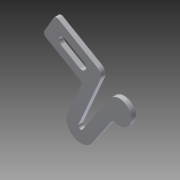
# Autodesk Inventor part: plastic-spring
Saved by Autodesk Inventor 2015 (Build 190159000, 159)
## iProperties
Created: 2014-10-04
Part Number: plastic-spring
Material: ABS Plastic
Document SubType Name: Modeling
Designer: Adam
Density: 1.06 g/cm^3
Appearance: Smooth - White
Author: Adam
Autodesk Inventor part; units mm, degrees
ref_plane "YZ Plane" through (0, 0, 0) normal (1, 0, 0) x (0, 1, 0)
ref_plane "XZ Plane" through (0, 0, 0) normal (0, 1, 0) x (-1, 0, 0)
ref_plane "Work Plane1" through (0, 0, 0.5) normal (0, 0, 1) x (1, 0, 0)
sketch "Sketch1" plane through (0, 0, 0.5) normal (0, 0, 1) x (1, 0, 0)
  line L0 (-82.7297, 47.8765) -> (82.7746, -47.6774) construction
  arc A0 (-7.7942, 4.6125) -> (-6.6121, 9.7651) centre (-15.5885, 9.1125) ccw construction
  arc A1 (-11.6654, 1.0125) -> (-7.7942, 4.6125) centre (-15.5885, 9.1125) ccw construction
  line L1 (-11.2583, 6.6125) -> (-15.5885, 9.1125) construction
  line L2 (-12.6807, 17.8261) -> (-21.6807, 2.2376) construction
  line L3 (-21.3116, 18.0806) -> (-26.3941, 9.2775) construction
  line L4 (-23.2429, 13.5318) -> (-25.2874, 14.7122) construction
  line L5 (-28.644, 9.9991) -> (-48.2897, 21.3415) construction
  line L6 (-42.5297, 31.3181) -> (-22.884, 19.9757) construction
  arc A2 (-28.7943, 15.1203) -> (-27.3943, 17.5452) centre (-28.0943, 16.3328) ccw construction
  line L7 (-27.3943, 17.5452) -> (-32.5904, 20.5452) construction
  arc A3 (-32.5904, 20.5452) -> (-33.9904, 18.1203) centre (-33.2904, 19.3328) ccw construction
  line L8 (-33.9904, 18.1203) -> (-28.7943, 15.1203) construction
  arc A4 (-13.829, 2.4121) -> (-16.4545, 9.6125) centre (-12.1244, 7.1125) ccw
  line L9 (-16.3046, 9.8558) -> (-30.232, -11.3665)
  line L10 (-20.1032, 14.7286) -> (-31.9722, -10.3906)
  arc A5 (-31.9722, -10.3906) -> (-30.232, -11.3665) centre (-31.068, -10.8179) ccw
  arc A6 (-20.1032, 14.7286) -> (-21.3157, 18.6083) centre (-22.8157, 16.0103) ccw
  arc A7 (-28.2563, 9.1773) -> (-28.6605, 10.4705) centre (-29.1605, 9.6045) ccw
  line L11 (-28.2563, 9.1773) -> (-36.4929, -8.2546)
  line L12 (-15.5944, 1.8249) -> (-26.0517, -14.1098)
  line L13 (-29.644, 8.267) -> (-28.644, 9.9991) construction
  line L14 (-15.2247, 16.6235) -> (-28.1306, -5.7301) construction
  arc A8 (-13.829, 2.4121) -> (-15.5944, 1.8249) centre (-14.3403, 1.0019) ccw
  arc A9 (-28.9943, 14.7739) -> (-27.1943, 17.8916) centre (-28.0943, 16.3328) ccw
  line L15 (-28.9943, 14.7739) -> (-36.7885, 19.2739)
  line L16 (-34.9885, 22.3916) -> (-27.1943, 17.8916)
  line L17 (-28.6605, 10.4705) -> (-43.3316, 18.9409)
  line L18 (-43.8807, 20.9899) -> (-40.0207, 27.6756)
  line L19 (-37.9717, 28.2247) -> (-21.3157, 18.6083)
  line L20 (-12.1244, 7.1125) -> (-15.5944, 1.8249) construction
  arc A10 (-36.4929, -8.2546) -> (-26.0517, -14.1098) centre (-31.068, -10.8179) ccw
  arc A11 (-34.9885, 22.3916) -> (-36.7885, 19.2739) centre (-35.8885, 20.8328) ccw
  arc A12 (-43.8807, 20.9899) -> (-43.3316, 18.9409) centre (-42.5816, 20.2399) ccw
  arc A13 (-37.9717, 28.2247) -> (-40.0207, 27.6756) centre (-38.7217, 26.9256) ccw
  point P0 (0, 0)
  point P1 (-31.0672, 39.9799)
  point P2 (-50.0597, 7.0838)
  dimension "d28" = 2
  dimension "d30" = 2
  dimension "d31" = 6
  dimension "d32" = 6
  dimension "d33" = 5
  dimension "d34" = 25
  dimension "d35" = 3
  dimension "d37" = 0.4
  dimension "d38" = 0.4
  dimension "d39" = 0.4
  dimension "d40" = 10
  dimension "d41" = 5
  dimension "d42" = 9
  dimension "d44" = 0.25
  dimension "d45" = 1.5
  constraints: 32 end point, 21 point on circle, 20 tangent, 10 centre point, 7 parallel, 4 point on line, 2 coincident, 2 collinear, 2 perpendicular, 1 equal radius, 3 other
  measures "d28" diameter of A5
  measures "d30" diameter of A7
  measures "d31" diameter of A6
  measures "d32" distance between parallel lines of L3 L14
  measures "d33" distance from line of A2.centre L3
  measures "d34" distance from line of L0 A5.centre
  measures "d35" diameter of A8
  measures "d37" distance between parallel lines of L16 L7
  measures "d38" distance between parallel lines of L6 L19
  measures "d39" distance between parallel lines of L17 L5
  measures "d40" distance from line of A3.centre L18
  measures "d41" radial gap between concentric circles of A10 A5
  measures "d42" distance of A2.centre A11.centre
  measures "d44" distance from line of L13 A7.centre
  measures "d45" radius of A12
extrude "Extrusion1" add sketch "Sketch1" along normal blind 2
equation "\"d39\" = d38"
body "Solid1"
